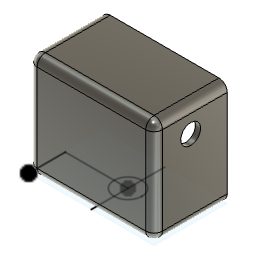
Open-Fluorometer-Main-Housing v4 (Autodesk Fusion 360 design; units mm, degrees)
Autodesk Fusion 360 part; units mm, degrees
note: some values were not read from the file. Set by a fixed rule: which sketch regions a step uses.
sketch "Sketch1" plane through (0, 0, 0) normal (0, 1, 0) x (1, 0, 0)
  line L0 (0, 0) -> (120, 0)
  line L1 (120, 0) -> (120, -100)
  line L2 (120, -100) -> (0, -100)
  line L3 (0, -100) -> (0, 0)
  dimension "d1" = 120
  dimension "d2" = 100
  constraint horizontal L0
  constraint vertical L1
  constraint horizontal L2
  constraint vertical L3
  constraint coincident L0.start L3.end
  measures "d1" distance of L0.start L0.end
  measures "d2" distance of L0.start L2.end
extrude "Extrude1" add sketch "Sketch1" along normal blind 70 makes body 1
shell "Shell1" thickness 5 removed faces 1 at (40, 70, 66.6667) on bodies 1
sketch "Sketch2" plane through (0, 0, 0) normal (0, 0, -1) x (1, 0, 0)
  line L0 (120, 0) -> (0, 0)
  line L1 (0, 0) -> (0, -70)
  line L2 (0, -70) -> (120, -70)
  line L3 (120, -70) -> (120, 0)
  line L4 (60, 0) -> (60, -70)
  line L5 (0, -35) -> (0, 0)
  line L6 (0, 0) -> (0, -35)
  line L7 (0, -35) -> (60, -35)
  circle A0 centre (60, -35) radius 13.25
  dimension "d6" = 26.5
  constraint midpoint L0 L4.start
  constraint midpoint L2 L4.end
  constraint midpoint L1 L5.start
  constraint coincident L0.end L1.start
  constraint midpoint L4 L7.end
  constraint coincident L7.end A0.centre
  measures "d6" diameter of A0
hole "Hole1" at (60, 35, 0) direction (0, 0, 1) diameter 27 depth 5 tip angle 180 bodies 1
sketch "Sketch3" plane through (0, 0, 0) normal (0, 0, -1) x (1, 0, 0)
  circle A0 centre (60, -35) radius 13.5
  line L0 (120, 0) -> (0, 0)
  line L1 (0, 0) -> (0, -70)
  line L2 (0, -70) -> (120, -70)
  line L3 (120, -70) -> (120, 0)
  line L4 (0, 0) -> (60, 0)
  line L5 (60, -70) -> (60, 0)
  line L6 (0, -35) -> (60, -35)
  line L7 (60, -35) -> (37.5, -35)
  circle A1 centre (37.5, -35) radius 1.25
  line L8 (37.5, -35) -> (82.5, -35)
  circle A2 centre (82.5, -35) radius 1.25
  dimension "d10" = 22.5
  dimension "d11" = 2.5
  dimension "d12" = 45
  dimension "d13" = 2.5
  constraint coincident L0.end L1.start
  constraint midpoint L0 L4.end
  constraint midpoint L2 L5.start
  constraint midpoint L1 L6.start
  constraint coincident A0.centre L6.end
  constraint perpendicular L5 L7
  constraint coincident L7.end A1.centre
  constraint parallel L6 L8
  constraint coincident L8.end A2.centre
  measures "d10" distance of A0.centre L7.end
  measures "d11" diameter of A1
  measures "d12" distance of L7.end L8.end
  measures "d13" diameter of A2
hole "Hole2" at (37.5, 35, 0) direction (0, 0, 1) diameter 2.5 depth 5 tip angle 180 bodies 1
sketch "Sketch4" plane through (0, 0, 0) normal (0, 1, 0) x (1, 0, 0)
hole "Hole3" at (82.5, 35, 0) direction (0, 0, 1) diameter 2.5 depth 5 tip angle 180 bodies 1
sketch "Sketch5" plane through (0, 5, 0) normal (0, 1, 0) x (-1, 0, 0)
  line L0 (-5, 95) -> (-115, 95)
  line L1 (-115, 95) -> (-115, 5)
  line L2 (-115, 5) -> (-5, 5)
  line L3 (-5, 5) -> (-5, 95)
  line L4 (-5, 5) -> (-9, 5)
  line L5 (-9, 5) -> (-9, 9)
  circle A0 centre (-9, 9) radius 4
  line L6 (-9, 9) -> (-111, 9)
  circle A1 centre (-111, 9) radius 4
  line L7 (-9, 9) -> (-9, 91)
  circle A2 centre (-9, 91) radius 4
  line L8 (-9, 91) -> (-111, 91)
  circle A3 centre (-111, 91) radius 4
  dimension "d20" = 4
  dimension "d21" = 4
  dimension "d22" = 8
  dimension "d23" = 102
  dimension "d24" = 8
  dimension "d25" = 82
  dimension "d26" = 8
  dimension "d27" = 102
  dimension "d28" = 8
  constraint coincident L2.end L3.start
  constraint perpendicular L3 L4
  constraint perpendicular L2 L5
  constraint coincident L5.end A0.centre
  constraint perpendicular L1 L6
  constraint coincident L6.end A1.centre
  constraint perpendicular L0 L7
  constraint coincident L7.end A2.centre
  constraint perpendicular L1 L8
  constraint coincident L8.end A3.centre
  measures "d20" distance of L2.end L4.end
  measures "d21" distance of L4.end L5.end
  measures "d22" diameter of A0
  measures "d23" distance of L5.end L6.end
  measures "d24" diameter of A1
  measures "d25" distance of L5.end L7.end
  measures "d26" diameter of A2
  measures "d27" distance of L7.end L8.end
  measures "d28" diameter of A3
extrude "Extrude2" add sketch "Sketch5" along normal blind 62.5 separate body contours A1 makes body 2
extrude "Extrude3" add sketch "Sketch5" along normal blind 62.5 separate body contours L5 A0 L7 | L5 A0 L6 | A0 L6 L7 makes body 3
extrude "Extrude4" add sketch "Sketch5" along normal blind 62.5 separate body contours L7 A2 L8 | L7 A2 L8 makes body 4
extrude "Extrude5" add sketch "Sketch5" along normal blind 62.5 separate body contours A3 makes body 5
sketch "Sketch6" plane through (120, 0, 0) normal (1, 0, 0) x (0, 1, 0)
  line L0 (0, 100) -> (0, 0)
  line L1 (0, 0) -> (70, 0)
  line L2 (70, 0) -> (70, 100)
  line L3 (70, 100) -> (0, 100)
  line L4 (0, 100) -> (0, 75)
  line L5 (0, 75) -> (35, 75)
  circle A0 centre (35, 75) radius 9.5
  dimension "d37" = 25
  dimension "d38" = 35
  dimension "d39" = 19
  constraint coincident L0.start L3.end
  constraint perpendicular L3 L4
  constraint perpendicular L2 L5
  constraint coincident L5.end A0.centre
  measures "d37" distance of L0.start L4.end
  measures "d38" distance of L4.end L5.end
  measures "d39" diameter of A0
hole "Hole4" at (120, 35, 75) direction (-1, 0, 0) diameter 19 depth 5 tip angle 180 bodies 1
sketch "Sketch7" plane through (0, 67.5, 0) normal (0, 1, 0) x (-1, 0, 0)
  circle A0 centre (-9, 9) radius 4
  circle A1 centre (-9, 9) radius 1.75
  dimension "d43" = 3.5
  constraint concentric A0 A1
  measures "d43" diameter of A1
fillet "Fillet1" radius 8 2 edges at (120, 35, 0) (0, 35, 0) on bodies 1
fillet "Fillet2" radius 8 2 edges at (0, 35, 100) (120, 35, 100) on bodies 1
fillet "Fillet3" radius 4 2 edges at (5, 37.5, 95) (115, 37.5, 95) on bodies 1
fillet "Fillet4" radius 4 2 edges at (5, 37.5, 5) (115, 37.5, 5) on bodies 1
fillet "Fillet5" radius 8 8 edges at (2.3431, 0, 97.6569) (0, 0, 50) (2.3431, 0, 2.3431) (60, 0, 0) (117.6569, 0, 2.3431) (120, 0, 50) (117.6569, 0, 97.6569) (60, 0, 100) on bodies 1
hole "Hole5" at (9, 67.5, 9) direction (0, -1, 0) diameter 3.5 depth 4 tip angle 180 bodies 3
hole "Hole6" at (111, 67.5, 9) direction (0, -1, 0) diameter 3.5 depth 4 tip angle 180 bodies 2
hole "Hole7" at (9, 67.5, 91) direction (0, -1, 0) diameter 3.5 depth 4 tip angle 180 bodies 4
hole "Hole8" at (111, 67.5, 91) direction (0, -1, 0) diameter 3.5 depth 4 tip angle 180 bodies 5
